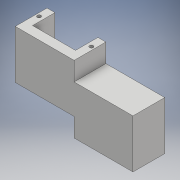
# Autodesk Inventor part: FEMUR
Saved by Autodesk Inventor 2017 (Build 210142000, 142)
## iProperties
Created: 2018-01-06
Part Number: FEMUR
Material: Generic
Document SubType Name: Modeling
Designer: Alex
Density: 1 g/cm^3
Appearance: Default
Author: Alex
Autodesk Inventor part; units mm, degrees
ref_plane "YZ Plane" through (0, 0, 0) normal (1, 0, 0) x (0, 1, 0)
ref_plane "XZ Plane" through (0, 0, 0) normal (0, 1, 0) x (-1, 0, 0)
ref_plane "XY Plane" through (0, 0, 0) normal (0, 0, 1) x (1, 0, 0)
sketch "Sketch1" plane through (0, 0, 0) normal (0, 1, 0) x (-1, 0, 0)
  line L0 (31.5, 18) -> (0, 18)
  line L1 (0, 18) -> (0, -8)
  line L2 (0, -8) -> (31.5, -8)
  line L3 (31.5, -8) -> (31.5, 18)
  line L4 (0, -25.2) -> (0, 25.2) projected
  line L5 (-31.5, -18) -> (0, -18)
  line L6 (0, -18) -> (0, 8)
  line L7 (0, 8) -> (-31.5, 8)
  line L8 (-31.5, 8) -> (-31.5, -18)
  point P0 (0, 0)
  dimension "d1" = 31.5
  dimension "d7" = 360
  dimension "d9" = 26
  dimension "d11" = 16
  constraints: 16 end point, 2 parallel, 1 collinear, 1 horizontal, 1 perpendicular, 17 other
  measures "d1" distance of L1.end L2.end
  measures "d9" distance of L2.end L0.start
  measures "d11" distance between parallel lines of L7 L2
extrude "Extrusion1" add sketch "Sketch1" along normal blind 17
sketch "Sketch3" plane through (0, 17, 0) normal (0, 1, 0) x (1, 0, 0)
  line L0 (-27.25, 3) -> (-4.25, 3)
  line L1 (-4.25, 3) -> (-4.25, -18)
  line L2 (-4.25, -18) -> (-27.25, -18)
  line L3 (-27.25, -18) -> (-27.25, 3)
  line L4 (27.25, -3) -> (4.25, -3)
  line L5 (4.25, -3) -> (4.25, 18)
  line L6 (4.25, 18) -> (27.25, 18)
  line L7 (27.25, 18) -> (27.25, -3)
  line L8 (0, 8) -> (-31.5, 8) projected
  line L9 (-31.5, -18) -> (0, -18) projected
  line L10 (-31.5, 8) -> (-31.5, -18) projected
  line L11 (0, -18) -> (0, -8) projected
  point P0 (0, 0)
  dimension "d16" = 360
  dimension "d18" = 5
  dimension "d19" = 4.25
  dimension "d20" = 4.25
  constraints: 16 end point, 2 parallel, 1 collinear, 1 horizontal, 1 perpendicular, 17 other
  measures "d18" distance between parallel lines of L0 L8
  measures "d19" distance between parallel lines of L10 L3
  measures "d20" distance between parallel lines of L11 L1
extrude "Extrusion2" cut sketch "Sketch3" against normal blind 12
sketch "Sketch4" plane through (-31.5, 0, 18) normal (0, 0, 1) x (1, 0, 0)
  circle A0 centre (1.75, 11) radius 1
  circle A1 centre (29.75, 11) radius 1
  line L0 (27.25, 17) -> (27.25, 5) projected
  line L1 (4.25, 5) -> (4.25, 17) projected
  point P0 (31.5, 0)
  point P1 (27.25, 11)
  dimension "d23" = 2
  dimension "d24" = 1.5
  dimension "d25" = 1.5
  constraints: 2 centre point, 2 horizontal alignment, 1 equal radius, 1 midpoint
  measures "d23" diameter of A1
  measures "d24" distance edge to line of A1 L0
  measures "d25" distance edge to line of A0 L1
extrude "Extrusion3" cut sketch "Sketch4" against normal blind 10
sketch "Sketch5" plane through (31.5, 0, -18) normal (0, 0, -1) x (-1, 0, 0)
  circle A0 centre (29.75, 11) radius 1
  circle A1 centre (1.75, 11) radius 1
  line L0 (27.25, 17) -> (27.25, 5) projected
  line L1 (4.25, 5) -> (4.25, 17) projected
  point P0 (31.5, 0)
  point P1 (27.25, 11)
  dimension "d26" = 1.5
  dimension "d27" = 1.5
  dimension "d28" = 2
  constraints: 2 centre point, 2 horizontal alignment, 1 equal radius, 1 midpoint
  measures "d26" distance edge to line of A1 L1
  measures "d27" distance edge to line of A0 L0
  measures "d28" diameter of A1
extrude "Extrusion4" cut sketch "Sketch5" against normal blind 10
equation "\"d1\" = servo_D"
equation "\"d9\" = servo_E + mat"
equation "\"d12\" = servo_B + mat"
equation "\"d18\" = mat"
equation "\"d19\" = -0.5 * servo_A + 0.5 * servo_D"
equation "\"d20\" = d19"
equation "\"d21\" = servo_B"
equation "\"d23\" = servo_H"
equation "\"d24\" = servo_L"
equation "\"d25\" = servo_L"
equation "\"d26\" = servo_L"
equation "\"d27\" = servo_L"
equation "\"d28\" = servo_H"
equation "\"mat\" = 5"
equation "\"servo_D\" = 31.5"
equation "\"servo_E\" = 21"
equation "\"servo_B\" = 12"
equation "\"servo_A\" = 23"
equation "\"servo_H\" = 2"
equation "\"servo_L\" = 1.5"
body "Solid1"
